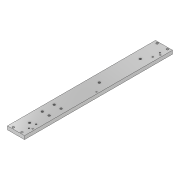
# Autodesk Inventor part: Lateral
Saved by Autodesk Inventor 2020 (Build 240168000, 168)
## iProperties
Created: 2020-05-08
Part Number: Lateral
Material: Aluminio 6061
Document SubType Name: Modeling
Designer: Pipi
Density: 2.7 g/cm^3
Appearance: Aluminum - Dark
Mass: 577.418 g
Surface Area: 548.393 cm^2
Volume: 213.858 cm^3
Author: Pipi
Autodesk Inventor part; units mm, degrees
ref_plane "YZ Plane" through (0, 0, 0) normal (1, 0, 0) x (0, 1, 0)
ref_plane "XZ Plane" through (0, 0, 0) normal (0, 1, 0) x (-1, 0, 0)
ref_plane "XY Plane" through (0, 0, 0) normal (0, 0, 1) x (1, 0, 0)
sketch "Boceto1" plane through (0, 0, 0) normal (0, 1, 0) x (-1, 0, 0)
  line L0 (22.6121, 129.278) -> (-27.3879, 129.278)
  line L1 (-27.3879, 129.278) -> (-27.3879, -304.722)
  line L2 (-27.3879, -304.722) -> (22.6121, -304.722)
  line L3 (22.6121, -304.722) -> (22.6121, 129.278)
  circle A0 centre (-15.3879, 104.278) radius 2
  circle A1 centre (-15.3879, 83.278) radius 2
  line L4 (-27.3879, -87.722) -> (-4.9043, -87.722)
  circle A2 centre (-15.3879, -279.722) radius 2
  circle A3 centre (-15.3879, -258.722) radius 2
  line L5 (-27.3879, -304.722) -> (-21.3879, -304.722)
  line L6 (-21.3879, -304.722) -> (-21.3879, -274.722)
  circle A4 centre (-21.3879, -274.722) radius 2
  circle A5 centre (-21.3879, -87.722) radius 2
  circle A6 centre (-21.3879, 99.278) radius 2
  circle A7 centre (-2.3879, -235.222) radius 3
  circle A8 centre (-2.3879, -115.222) radius 3
  circle A9 centre (-2.3879, 89.278) radius 3
  dimension "d4" = 434
  dimension "d5" = 50
  dimension "d16" = 4
  dimension "d17" = 4
  dimension "d18" = 25
  dimension "d19" = 21
  dimension "d20" = 12
  dimension "d21" = 12
  dimension "d85" = 12
  dimension "d86" = 12
  dimension "d87" = 21
  dimension "d89" = 30
  dimension "d90" = 4
  dimension "d91" = 4
  dimension "d92" = 44
  dimension "d93" = 44
  dimension "d94" = 217
  dimension "d95" = 6
  dimension "d96" = 25
  dimension "d97" = 69.5
  dimension "d98" = 6
  dimension "d99" = 120
  dimension "d100" = 25
  dimension "d101" = 6
  dimension "d102" = 25
  dimension "d103" = 40
  constraints: 14 end point, 10 centre point, 4 perpendicular, 4 symmetric about line, 2 coincident, 2 horizontal, 1 midpoint, 1 point on line, 3 other
  measures "d4" distance of L0.end L1.end
  measures "d5" distance of L0.start L0.end
  measures "d16" diameter of A0
  measures "d17" diameter of A1
  measures "d18" distance from line of L0 A0.centre
  measures "d19" distance of A0.centre A1.centre
  measures "d20" distance from line of L1 A0.centre
  measures "d21" distance from line of L1 A1.centre
  measures "d85" distance from line of L1 A2.centre
  measures "d86" distance from line of L1 A3.centre
  measures "d87" distance of A3.centre A2.centre
  measures "d89" distance of L5.end L6.end
  measures "d90" diameter of A4
  measures "d91" diameter of A5
  measures "d92" distance between parallel lines of L6 L3
  measures "d93" distance from line of L3 A5.centre
  measures "d94" distance from line of L2 A5.centre
  measures "d95" diameter of A7
  measures "d96" distance from line of L1 A7.centre
  measures "d97" distance from line of L2 A7.centre
  measures "d98" diameter of A8
  measures "d99" distance of A8.centre A7.centre
  measures "d100" distance from line of L1 A8.centre
  measures "d101" diameter of A9
  measures "d102" distance from line of L1 A9.centre
  measures "d103" distance from line of L0 A9.centre
extrude "Extrusión1" add sketch "Boceto1" along normal blind 10
sketch "Boceto2" plane through (0, 10, 0) normal (0, 1, 0) x (1, 0, 0)
  line L0 (-22.6121, -129.278) -> (27.3879, -129.278) projected
  line L1 (-22.6121, -129.278) -> (-22.6121, -124.278)
  line L2 (-22.6121, 304.722) -> (-22.6121, -129.278) projected
  line L3 (-22.6121, -124.278) -> (27.3879, -124.278)
  line L4 (27.3879, -129.278) -> (27.3879, 304.722) projected
  line L5 (27.3879, 304.722) -> (-22.6121, 304.722) projected
  line L6 (-22.6121, 304.722) -> (-22.6121, 299.722)
  line L7 (-22.6121, 299.722) -> (27.3879, 299.722)
  line L8 (-22.6121, -124.278) -> (-10.1121, -124.278)
  line L9 (27.3879, 299.722) -> (17.3879, 299.722)
  circle A0 centre (-10.1121, -124.278) radius 3
  circle A1 centre (14.8879, -124.278) radius 3
  circle A2 centre (-12.6121, 299.722) radius 3
  circle A3 centre (17.3879, 299.722) radius 3
  dimension "d6" = 5
  dimension "d7" = 5
  dimension "d8" = 12.5
  dimension "d9" = 10
  dimension "d10" = 6
  dimension "d11" = 6
  dimension "d12" = 6
  dimension "d13" = 6
  dimension "d30" = 5
  dimension "d74" = 5
  dimension "d110" = 10
  constraints: 12 end point, 5 point on line, 4 centre point, 2 coincident, 2 perpendicular
  measures "d6" distance of L0.start L1.end
  measures "d7" distance of L2.start L6.end
  measures "d8" distance of L1.end L8.end
  measures "d9" distance of L7.end L9.end
  measures "d10" diameter of A0
  measures "d11" diameter of A1
  measures "d12" diameter of A2
  measures "d13" diameter of A3
  measures "d30" distance from line of L0 A1.centre
  measures "d74" distance from line of L5 A2.centre
  measures "d110" distance of L6.end A2.centre
extrude "Extrusión2" cut sketch "Boceto2" against normal blind 20 contours A0 L3 | L3 A0 | A1 L3 | L3 A1 | A2 L7 | L7 A2 | A3 L7 | L7 A3
thread "Thread1" size "M4x0.7" class "6H" standard "ANSI Metric M Profile" length 40
thread "Thread2" size "M4x0.7" class "6H" standard "ANSI Metric M Profile" length 40
sketch "Boceto3" plane through (0, 0, 0) normal (0, -1, 0) x (1, 0, 0)
  line L0 (27.3879, 129.278) -> (27.3879, -304.722) projected
  line L1 (12.3879, 42.078) -> (-7.6121, 42.078)
  line L2 (-7.6121, 42.078) -> (-7.6121, 7.078)
  line L3 (-7.6121, 7.078) -> (12.3879, 7.078)
  line L4 (12.3879, 7.078) -> (12.3879, 42.078)
  circle A0 centre (12.3879, 7.078) radius 3
  circle A1 centre (-7.6121, 7.078) radius 3
  circle A2 centre (12.3879, 42.078) radius 3
  circle A3 centre (-7.6121, 42.078) radius 3
  line L5 (-22.6121, 129.278) -> (27.3879, 129.278) projected
  line L6 (-22.6121, -304.722) -> (-22.6121, 129.278) projected
  point P0 (-14161.5164, 17179.1084)
  point P1 (-14161.5164, 17617.1084)
  point P2 (-14211.5164, 17617.1084)
  point P3 (-14211.5164, 17179.1084)
  dimension "d58" = 35
  dimension "d59" = 15
  dimension "d60" = 87.2
  dimension "d61" = 15
  dimension "d62" = 20
  constraints: 8 end point, 4 centre point, 4 coincident, 3 other
  measures "d58" distance of L3.end L1.start
  measures "d62" distance between parallel lines of L2 L4
hole "Agujero1" at (12.3879, 0, 42.078) at (-7.6121, 0, 42.078) at (12.3879, 0, 7.078) at (-7.6121, 0, 7.078) direction (0, 1, 0) diameter 6 depth 12 tip angle 118
thread "Rosca5" size "M4x0.7" class "6H" standard "ISO Metric profile" length 430
thread "Rosca6" size "M4x0.7" class "6H" standard "ISO Metric profile" length 430
thread "Rosca7" size "M6x1" class "6H" standard "ISO Metric profile" length 430
thread "Rosca8" size "M6x1" class "6H" standard "ISO Metric profile" length 430
thread "Rosca9" size "M6x1" class "6H" standard "ISO Metric profile" length 430
thread "Rosca10" size "M6x1" class "6H" standard "ISO Metric profile" length 430
thread "Rosca11" size "M4x0.7" class "6H" standard "ISO Metric profile" length 430
thread "Rosca12" size "M6x1" class "6H" standard "ISO Metric profile" length 100
thread "Rosca13" size "M6x1" class "6H" standard "ISO Metric profile" length 100
thread "Rosca14" size "M6x1" class "6H" standard "ISO Metric profile" length 100
equation "\"d100\" = d96"
equation "\"d102\" = d96"
equation "\"d110\" = d9"
